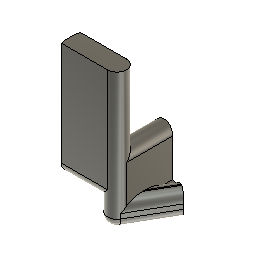
pen goliath cartridge v5 (Autodesk Fusion 360 archive; units mm, degrees)
design "bolt path"
Autodesk Fusion 360 part; units mm, degrees
sketch "Sketch1" plane through (0, 0, 0) normal (0, 0, 1) x (1, 0, 0)
  circle A0 centre (0, 0) radius 5
  line L0 (-1, 4.898979) -> (-1, 0)
  line L1 (1, 4.898979) -> (1, 0)
  line L2 (-1, 0) -> (1, 0)
  line L3 (1.583464, 4.742641) -> (-0.57735, 1)
  arc A1 (-1, 3.872983) -> (2.802517, 2.854102) centre (0, 0) ccw
  line L4 (-0.866025, 0.5) -> (0.866025, -0.5)
  line L5 (0.866025, -0.5) -> (3.315515, 3.742641)
  circle A2 centre (0, 0) radius 1
  line L6 (0, -1) -> (-4.898979, -1)
  line L7 (0, 1) -> (-4.898979, 1)
  dimension "d1" = 10
  dimension "d2" = 2
  dimension "d3" = 8
  dimension "d4" = 2
  dimension "d24" = 30
  constraint coincident A0.centre A1.centre
  constraint vertical L0
  constraint vertical L1
  constraint horizontal L2
  constraint midpoint A0.centre L2
  constraint perpendicular L3 L4
  constraint midpoint A0.centre L4
  constraint perpendicular L4 L5
  constraint coincident L0.end A2
  constraint coincident A2 L6.start
  constraint tangent A2 L6
  constraint horizontal L6
  constraint coincident A2 L7.start
  constraint tangent A2 L7
  constraint perpendicular L0 L7
  constraint tangent L3 A2
  measures "d1" diameter of A0
  measures "d2" distance of L0 L1
  measures "d3" diameter of A1
  measures "d24" angle of L1 L5
extrude "Extrude1" add sketch "Sketch1" along normal blind 4.5 and the other way blind 1 contours A0 L0 L1 L3 L7 | L1 L3 A2 L7 | L2 L4 A2 | L2 L4 A2 | L2 L4 A2 | L0 A2 L7 | L2 L4 A2 picked at (-0.19245, 2.868345) picked at (0.140883, 1.910684) picked at (0.549286, -0.374497) picked at (0.663815, -0.043509) picked at (-0.332401, 0.575736) picked at (-0.752508, 0.911017) picked at (-0.663815, 0.043509)
extrude "Extrude2" add sketch "Sketch1" against normal blind 2.5 contours A0 L1 L3 L5 A2 picked at (1.600839, 2.195384)
extrude "Extrude3" add 1 faces at (-0.333333, 2.87701, -1) along direction (0, 0, -1) up to surface (1.5 mm away)
extrude "Extrude4" add sketch "Sketch1" along normal blind 2 from surface at -2.5 contours A0 L1 L3 picked at (1.195888, 4.463116)
extrude "Extrude5" add sketch "Sketch1" along normal blind 2 contours A0 A1 L6 L7 | A0 L0 A1 L7 | L0 A1 A2 L6 L7 | L0 A1 L7 picked at (-4.659161, 0) picked at (-4.491108, 1.23404) picked at (-1.957661, 0.666667) picked at (-2.335795, 2.085411)
extrude "Extrude6" add sketch "Sketch1" along normal blind 10 from surface at 2 contours A0 A1 L6 L7 | L0 A1 A2 L6 L7 | L2 L4 A2 | L2 L4 A2 | L2 L4 A2 | L0 A2 L7 | L2 L4 A2 picked at (-4.659161, 0) picked at (-1.957661, 0.666667) picked at (0.549286, -0.374497) picked at (0.663815, -0.043509) picked at (-0.332401, 0.575736) picked at (-0.752508, 0.911017) picked at (-0.663815, 0.043509)
fillet "Fillet1" radius 1 8 edges at (2.09077, 1.62132, 0) (2.09077, 1.62132, -2.5) (1.291732, 4.237346, 0) (-1, 2.94949, 4.5) (-1, 2.44949, -2.5) (1, 2.44949, 4.5) (-0.258819, -0.965926, -2.5) (-2.44949, -1, 0)

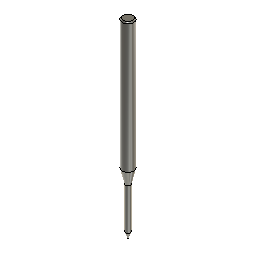
design "pen cartridege"
Autodesk Fusion 360 part; units mm, degrees
sketch "Sketch1" plane through (0, 0, 0) normal (0, 0, 1) x (1, 0, 0)
  circle A0 centre (0, 0) radius 1.25
  circle A1 centre (0, 0) radius 2.9
  dimension "d1" = 2.5
  dimension "d2" = 5.8
  constraint coincident A0.centre A1.centre
  measures "d1" diameter of A0
  measures "d2" diameter of A1
extrude "Extrude1" add sketch "Sketch1" along normal blind 95.9 contours A0 | A1
extrude "Extrude2" cut sketch "Sketch1" along normal blind 23.7
chamfer "Chamfer1" distance 1 distance2 3 1 edges at (-1.1654, 0.452, 0) measured on face at (-0.4866, 0.4642, 0)
chamfer "Chamfer2" distance 7 distance2 1.65 1 edges at (-2.7037, -1.0487, 23.7) measured on face at (2.8856, -0.2887, 47.7667)
chamfer "Chamfer3" distance 0.6 angle 45 1 edges at (-2.7037, -1.0487, 95.9)
sketch "Sketch2" plane through (0, 0, 0) normal (1, 0, 0) x (0, 1, 0)
  line L0 (-1.25, 3) -> (1.25, 3)
  line L1 (1.25, 3) -> (5, 13.303)
  line L2 (5, 13.303) -> (-5, 13.303) construction
  line L3 (0, 13.303) -> (0, 0)
  dimension "d13" = 10
  dimension "d14" = 70
  constraint coincident L0 L1.start
  constraint horizontal L2
  constraint midpoint L2 L3.start
  constraint coincident L3.end origin
  constraint vertical L3
  constraint coincident L0.end L1.start
  measures "d13" distance of L1.end L2.end
  measures "d14" angle of L1 L2
